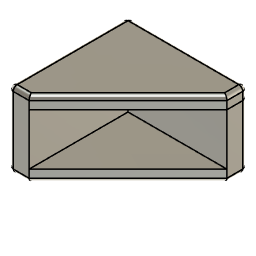
Base Bracket v7 (Autodesk Fusion 360 design; units mm, degrees)
Autodesk Fusion 360 part; units mm, degrees
sketch "Sketch1" plane through (0, 0, 0) normal (0, 0, 1) x (1, 0, 0)
  line L0 (0, 0) -> (0, 25)
  line L1 (0, 25) -> (25, 25)
  line L2 (25, 25) -> (25, 25)
  line L3 (25, 25) -> (25, 30)
  line L4 (25, 30) -> (25, 30)
  line L5 (25, 30) -> (25, 25)
  line L6 (0, 0) -> (-5, 0)
  line L7 (-5, 0) -> (-5, 30)
  line L8 (-5, 30) -> (25, 30)
  line L9 (25, 25) -> (0, 0)
  dimension "d1" = 25
  dimension "d2" = 25
  dimension "d3" = 5
  dimension "d4" = 5
  constraint coincident L0.start L6.start
  constraint vertical L0
  constraint perpendicular L0 L1
  constraint vertical L3
  constraint vertical L5
  constraint perpendicular L0 L6
  constraint perpendicular L6 L7
  measures "d1" distance of L0.start L0.end
  measures "d2" distance of L0.end L1.end
  measures "d3" distance of L1.end L3.end
  measures "d4" distance of L0.start L6.end
extrude "Extrude1" add sketch "Sketch1" against normal blind 3
extrude "Extrude2" add sketch "Sketch1" along normal blind 13 contours L0 L1 L3 L5 L6 L7 L8
sketch "Sketch2" plane through (0, 0, 13) normal (0, 0, 1) x (-1, 0, 0)
  line L0 (0, 0) -> (0, -25)
  line L1 (0, -25) -> (-25, -25)
  line L2 (-25, -25) -> (-25, -30)
  line L3 (-25, -30) -> (5, -30)
  line L4 (5, -30) -> (5, 0)
  line L5 (5, 0) -> (0, 0)
  line L6 (-25, -25) -> (0, 0)
  constraint coincident L1.end L2.start
  constraint coincident L0.start L5.end
extrude "Extrude3" add sketch "Sketch2" along normal blind 3
fillet "Fillet1" radius 1 10 edges at (-2.5, 0, -3) (12.5, 12.5, -3) (25, 27.5, -3) (10, 30, -3) (-5, 15, -3) (-2.5, 0, 16) (12.5, 12.5, 16) (25, 27.5, 16) (-5, 15, 16) (10, 30, 16)
fillet "Fillet2" radius 1 3 edges at (-4.7071, 29.7071, -2.7071) (-5, 30, 6.5) (-4.7071, 29.7071, 15.7071)
fillet "Fillet3" radius 1 7 edges at (24.7071, 29.7071, -2.7071) (25, 30, 5.5) (25, 30, 14) (24.7071, 29.7071, 15.7071) (-4.7071, 0.2929, -2.7071) (-5, 0, 6.5) (-4.7071, 0.2929, 15.7071)
